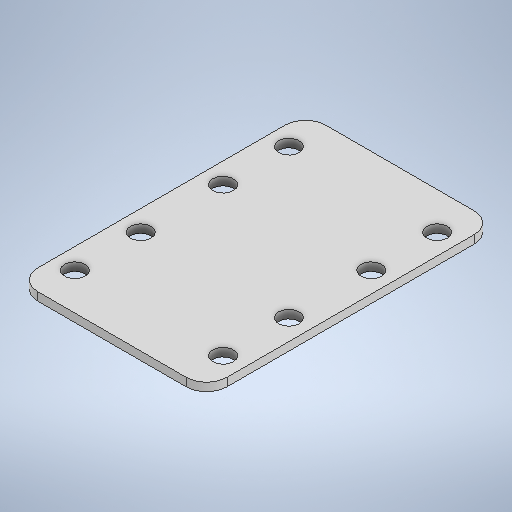
# Autodesk Inventor part: 17
Saved by Autodesk Inventor 2025.1 (Build 291241000, 241)
## iProperties
Created: 2024-09-12
Part Number: 17
Material: Generic
Document SubType Name: Sheet Metal
Designer: ffogue
Density: 1 g/cm^3
Sheet Metal Rule: Default_mm
Appearance: Default
Author: ffogue
Autodesk Inventor part; units mm, degrees
ref_plane "YZ Plane" through (0, 0, 0) normal (1, 0, 0) x (0, 1, 0)
ref_plane "XZ Plane" through (0, 0, 0) normal (0, 1, 0) x (-1, 0, 0)
ref_plane "XY Plane" through (0, 0, 0) normal (0, 0, 1) x (1, 0, 0)
sketch "Sketch1" plane through (0, 0, 0) normal (0, 0, 1) x (1, 0, 0)
  line L0 (-11.5, -17.5) -> (11.5, -17.5)
  line L1 (11.5, -17.5) -> (11.5, 17.5)
  line L2 (11.5, 17.5) -> (-11.5, 17.5)
  line L3 (-11.5, 17.5) -> (-11.5, -17.5)
  line L4 (-11.5, -17.5) -> (11.5, 17.5) construction
  line L5 (11.5, -17.5) -> (-11.5, 17.5) construction
  point P0 (0, 0)
  dimension "d0" = 23
  dimension "d1" = 35
  measures "d0" distance of L1.end L2.end
  measures "d1" distance of L2.end L0.start
extrude "Plate1" add sketch "Sketch1" along normal blind 1
sketch "Sketch2" plane through (0, 0, 1) normal (0, 0, 1) x (1, 0, 0)
  line L0 (-11.5, -17.5) -> (-11.5, 17.5) projected
  point P0 (0, 0)
  point P1 (-9, -13)
  point P2 (9, -13)
  point P3 (-9, -5)
  point P4 (9, -5)
  dimension "d3" = 18
  dimension "d4" = 9
  dimension "d5" = 8
  dimension "d8" = 2.5
  dimension "d17" = 5
  constraints: 2 horizontal alignment, 2 vertical alignment
  measures "d3" distance of point (9, -13) point (-9, -13)
  measures "d4" horizontal distance of point (0, 0) point (-9, -13)
  measures "d5" distance of point (9, -5) point (9, -13)
  measures "d8" distance from line of L0 point (-9, -13)
  measures "d17" vertical distance of point (0, 0) point (-9, -5)
hole "Hole1" at (-9, -13, 1) at (9, -13, 1) at (-9, -5, 1) at (9, -5, 1) direction (0, 0, -1) diameter 2.5 depth 1
fillet "Fillet1" radius 2.5 4 edges at (11.5, 17.5, 0.5) (11.5, -17.5, 0.5) (-11.5, -17.5, 0.5) (-11.5, 17.5, 0.5)
mirror "Mirror1" about plane through (0, 0, 0) normal (0, 1, 0) of "Hole1"
equation "\"d4\" = 0.5 * d3"
equation "\"d14\" = Stärke"
equation "\"d2\" = Stärke"
equation "\"Biegeradius\" = Stärke"
equation "\"BreiteBiegungsfreistellung\" = Stärke"
equation "\"TiefeBiegungsfreistellung\" = 0.5 * Stärke"
equation "\"GrößeEckenfreistellung\" = 4 * Stärke"
equation "\"MinimalRest\" = 2 * Stärke"
equation "\"Übergangsradius\" = Biegeradius"
equation "\"JacobiRadiusGröße\" = Biegeradius"
equation "\"Abstandsgröße\" = Stärke"
equation "\"Stärke\" = 1"
body "Solid1"
